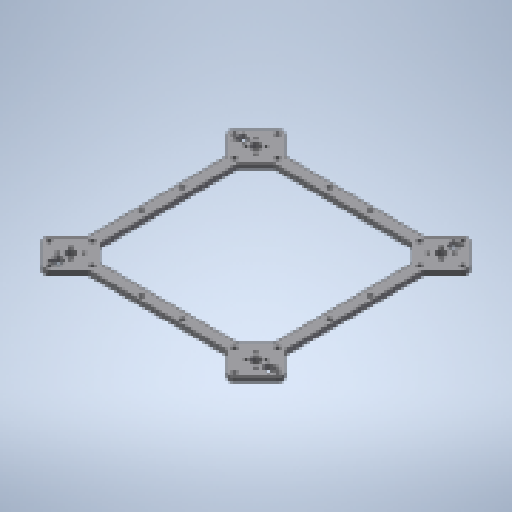
# Autodesk Inventor part: 终版
Saved by Autodesk Inventor 2025.2 (Build 292293000, 293)
## iProperties
Created: 2025-10-21
Part Number: 终版
Material: 常规
Document SubType Name: Modeling
Designer: BO‘S_SLAVE
Density: 1 g/cm^3
Appearance: 默认
Author: BO‘S_SLAVE
Autodesk Inventor part; units mm, degrees
ref_plane "YZ Plane" through (0, 0, 0) normal (1, 0, 0) x (0, 1, 0)
ref_plane "XZ Plane" through (0, 0, 0) normal (0, 1, 0) x (-1, 0, 0)
ref_plane "XY Plane" through (0, 0, 0) normal (0, 0, 1) x (1, 0, 0)
sketch "草图1" plane through (0, 0, 0) normal (0, 1, 0) x (-1, 0, 0)
  line L0 (0, 0) -> (-155.5635, 0)
  line L1 (-155.5635, 0) -> (-155.5635, -155.5635)
  line L2 (-155.5635, -155.5635) -> (0, -155.5635)
  line L3 (0, -155.5635) -> (0, 0)
  line L4 (0, 0) -> (-155.5635, -155.5635)
  line L5 (0, -155.5635) -> (-155.5635, 0)
  line L6 (5, 5) -> (-160.5635, 5)
  line L7 (-160.5635, 5) -> (-160.5635, -160.5635)
  line L8 (-160.5635, -160.5635) -> (5, -160.5635)
  line L9 (5, -160.5635) -> (5, 5)
  line L10 (-5, -5) -> (-150.5635, -5)
  line L11 (-150.5635, -5) -> (-150.5635, -150.5635)
  line L12 (-150.5635, -150.5635) -> (-5, -150.5635)
  line L13 (-5, -150.5635) -> (-5, -5)
  line L14 (0, 24.7487) -> (-24.7487, 0)
  line L15 (24.7487, 0) -> (0, 24.7487)
  line L16 (0, -24.7487) -> (24.7487, 0)
  line L17 (0, -24.7487) -> (-24.7487, 0)
  circle A0 centre (-94.7817, 1.109) radius 1.65
  circle A1 centre (-60.7817, 1.109) radius 1.65
  line L18 (0, -24.7487) -> (0, 24.7487)
  line L19 (-77.7817, -5) -> (-77.7817, 5)
  circle A2 centre (0, 0) radius 3.5
  circle A3 centre (-5.6569, -5.6569) radius 1.15
  circle A4 centre (5.6569, 5.6569) radius 1.15
  circle A5 centre (-4.2426, 4.2426) radius 1.15
  circle A6 centre (4.2426, -4.2426) radius 1.15
  line L20 (5.6569, 5.6569) -> (0, 0)
  line L21 (4.2426, -4.2426) -> (-4.2426, 4.2426)
  circle A7 centre (18, 0) radius 1.65
  line L22 (24.7487, 0) -> (0, 0)
  circle A8 centre (0, 18) radius 1.65
  circle A9 centre (-18, 0) radius 1.65
  circle A10 centre (0, -18) radius 1.65
  line L23 (-155.5635, 24.7487) -> (-180.3122, 0)
  line L24 (-130.8148, 0) -> (-155.5635, 24.7487)
  line L25 (-130.8148, 0) -> (-155.5635, -24.7487)
  line L26 (-180.3122, 0) -> (-155.5635, -24.7487)
  circle A11 centre (-173.5635, 0) radius 1.65
  circle A12 centre (-155.5635, 18) radius 1.65
  circle A13 centre (-137.5635, 0) radius 1.65
  circle A14 centre (-155.5635, -18) radius 1.65
  circle A15 centre (-159.8061, -4.2426) radius 1.15
  circle A16 centre (-151.3209, 4.2426) radius 1.15
  circle A17 centre (-161.2203, 5.6569) radius 1.15
  circle A18 centre (-155.5635, 0) radius 3.5
  circle A19 centre (-149.9066, -5.6569) radius 1.15
  line L27 (-180.3122, -155.5635) -> (-155.5635, -180.3122)
  line L28 (-155.5635, -130.8148) -> (-180.3122, -155.5635)
  line L29 (-155.5635, -130.8148) -> (-130.8148, -155.5635)
  line L30 (-155.5635, -180.3122) -> (-130.8148, -155.5635)
  circle A20 centre (-155.5635, -173.5635) radius 1.65
  circle A21 centre (-173.5635, -155.5635) radius 1.65
  circle A22 centre (-155.5635, -137.5635) radius 1.65
  circle A23 centre (-137.5635, -155.5635) radius 1.65
  circle A24 centre (-151.3209, -159.8061) radius 1.15
  circle A25 centre (-159.8061, -151.3209) radius 1.15
  circle A26 centre (-161.2203, -161.2203) radius 1.15
  circle A27 centre (-155.5635, -155.5635) radius 3.5
  circle A28 centre (-149.9066, -149.9066) radius 1.15
  line L31 (0, -180.3122) -> (24.7487, -155.5635)
  line L32 (-24.7487, -155.5635) -> (0, -180.3122)
  line L33 (-24.7487, -155.5635) -> (0, -130.8148)
  line L34 (24.7487, -155.5635) -> (0, -130.8148)
  circle A29 centre (18, -155.5635) radius 1.65
  circle A30 centre (0, -173.5635) radius 1.65
  circle A31 centre (-18, -155.5635) radius 1.65
  circle A32 centre (0, -137.5635) radius 1.65
  circle A33 centre (4.2426, -151.3209) radius 1.15
  circle A34 centre (-4.2426, -159.8061) radius 1.15
  circle A35 centre (5.6569, -161.2203) radius 1.15
  circle A36 centre (0, -155.5635) radius 3.5
  circle A37 centre (-5.6569, -149.9066) radius 1.15
  circle A38 centre (-156.6725, -94.7817) radius 1.65
  circle A39 centre (-156.6725, -60.7817) radius 1.65
  circle A40 centre (-60.7817, -156.6725) radius 1.65
  circle A41 centre (-94.7817, -156.6725) radius 1.65
  circle A42 centre (1.109, -60.7817) radius 1.65
  circle A43 centre (1.109, -94.7817) radius 1.65
  circle A44 centre (-60.7817, 1.1093) radius 1.65 projected
  circle A45 centre (-41.7817, -60.7817) radius 1.65 construction
  line L35 (-66.2817, -48.8909) -> (-66.2817, -106.6726) construction
  line L36 (-65.8148, -48.8909) -> (-66.2817, -48.8909) construction
  line L37 (-48.8909, -65.8148) -> (-65.8148, -48.8909) construction
  line L38 (-48.8909, -89.7487) -> (-48.8909, -65.8148) construction
  line L39 (-65.8148, -106.6726) -> (-48.8909, -89.7487) construction
  line L40 (-66.2817, -106.6726) -> (-65.8148, -106.6726) construction
  arc A46 (-61.6726, -28.8363) -> (-64.6726, -25.8363) centre (-64.6726, -28.8363) ccw construction
  line L41 (-61.6726, -35.8909) -> (-61.6726, -28.8363) construction
  arc A47 (-64.6726, -38.8909) -> (-61.6726, -35.8909) centre (-64.6726, -35.8909) ccw construction
  line L42 (-90.8909, -38.8909) -> (-64.6726, -38.8909) construction
  arc A48 (-93.8909, -35.8909) -> (-90.8909, -38.8909) centre (-90.8909, -35.8909) ccw construction
  line L43 (-93.8909, -28.8363) -> (-93.8909, -35.8909) construction
  arc A49 (-90.8909, -25.8363) -> (-93.8909, -28.8363) centre (-90.8909, -28.8363) ccw construction
  line L44 (-64.6726, -25.8363) -> (-90.8909, -25.8363) construction
  arc A50 (-115.3828, -60.3828) -> (-114.1807, -59.1807) centre (-113.7817, -60.7817) ccw construction
  line L45 (-114.1807, -59.1807) -> (-115.3828, -60.3828) construction
  circle A51 centre (-94.7817, -113.7817) radius 1.65 construction
  circle A52 centre (-155.5635, -137.5635) radius 1.65 construction
  line L46 (-157.9654, -162.7302) -> (-160.0223, -170.4065) construction
  line L47 (-153.1616, -162.7302) -> (-157.9654, -162.7302) construction
  line L48 (-151.1047, -170.4065) -> (-153.1616, -162.7302) construction
  line L49 (-160.0223, -170.4065) -> (-151.1047, -170.4065) construction
  circle A53 centre (-155.5635, -173.5635) radius 1.65 construction
  circle A54 centre (-137.5635, -155.5635) radius 1.65 construction
  circle A55 centre (-173.5635, -155.5635) radius 1.65 construction
  circle A56 centre (-151.3209, -159.8061) radius 1.15 construction
  circle A57 centre (-159.8061, -151.3209) radius 1.15 construction
  circle A58 centre (-161.2203, -161.2203) radius 1.15 construction
  arc A59 (-108.4906, -39.5876) -> (-107.7835, -37.8805) centre (-108.4906, -38.5876) ccw construction
  line L50 (-112.7333, -39.5876) -> (-108.4906, -39.5876) construction
  arc A60 (-113.4404, -39.2947) -> (-112.7333, -39.5876) centre (-112.7333, -38.5876) ccw construction
  line L51 (-115.683, -37.052) -> (-113.4404, -39.2947) construction
  arc A61 (-115.9759, -36.3449) -> (-115.683, -37.052) centre (-114.9759, -36.3449) ccw construction
  line L52 (-115.9759, -32.1023) -> (-115.9759, -36.3449) construction
  arc A62 (-114.2688, -31.3952) -> (-115.9759, -32.1023) centre (-114.9759, -32.1023) ccw construction
  line L53 (-107.7835, -37.8805) -> (-114.2688, -31.3952) construction
  arc A63 (-126.6328, -21.4454) -> (-125.9257, -19.7383) centre (-126.6328, -20.4454) ccw construction
  line L54 (-130.8754, -21.4454) -> (-126.6328, -21.4454) construction
  arc A64 (-131.5825, -21.1525) -> (-130.8754, -21.4454) centre (-130.8754, -20.4454) ccw construction
  line L55 (-133.8252, -18.9099) -> (-131.5825, -21.1525) construction
  arc A65 (-134.1181, -18.2028) -> (-133.8252, -18.9099) centre (-133.1181, -18.2028) ccw construction
  line L56 (-134.1181, -13.9602) -> (-134.1181, -18.2028) construction
  arc A66 (-132.4109, -13.253) -> (-134.1181, -13.9602) centre (-133.1181, -13.9602) ccw construction
  line L57 (-125.9257, -19.7383) -> (-132.4109, -13.253) construction
  arc A67 (-136.1181, -9.9602) -> (-136.4109, -9.253) centre (-137.1181, -9.9602) ccw construction
  line L58 (-136.1181, -14.2028) -> (-136.1181, -9.9602) construction
  arc A68 (-137.8252, -14.9099) -> (-136.1181, -14.2028) centre (-137.1181, -14.2028) ccw construction
  line L59 (-141.7749, -10.9602) -> (-137.8252, -14.9099) construction
  line L60 (-138.2394, -7.4246) -> (-141.7749, -10.9602) construction
  line L61 (-136.4109, -9.253) -> (-138.2394, -7.4246) construction
  arc A69 (-21.7383, -18.9099) -> (-21.4454, -18.2028) centre (-22.4454, -18.2028) ccw construction
  line L62 (-23.981, -21.1525) -> (-21.7383, -18.9099) construction
  arc A70 (-24.6881, -21.4454) -> (-23.981, -21.1525) centre (-24.6881, -20.4454) ccw construction
  line L63 (-28.9307, -21.4454) -> (-24.6881, -21.4454) construction
  arc A71 (-29.6378, -19.7383) -> (-28.9307, -21.4454) centre (-28.9307, -20.4454) ccw construction
  line L64 (-23.1525, -13.253) -> (-29.6378, -19.7383) construction
  arc A72 (-21.4454, -13.9602) -> (-23.1525, -13.253) centre (-22.4454, -13.9602) ccw construction
  line L65 (-21.4454, -18.2028) -> (-21.4454, -13.9602) construction
  arc A73 (-37.5876, -127.4612) -> (-37.2947, -128.1683) centre (-36.5876, -127.4612) ccw construction
  line L66 (-37.5876, -123.2186) -> (-37.5876, -127.4612) construction
  arc A74 (-35.8805, -122.5115) -> (-37.5876, -123.2186) centre (-36.5876, -123.2186) ccw construction
  line L67 (-27.981, -130.4109) -> (-35.8805, -122.5115) construction
  arc A75 (-28.6881, -132.1181) -> (-27.981, -130.4109) centre (-28.6881, -131.1181) ccw construction
  line L68 (-32.9307, -132.1181) -> (-28.6881, -132.1181) construction
  arc A76 (-33.6378, -131.8252) -> (-32.9307, -132.1181) centre (-32.9307, -131.1181) ccw construction
  line L69 (-37.2947, -128.1683) -> (-33.6378, -131.8252) construction
  arc A77 (-37.8805, -107.7835) -> (-39.5876, -108.4906) centre (-38.5876, -108.4906) ccw construction
  line L70 (-31.3952, -114.2688) -> (-37.8805, -107.7835) construction
  arc A78 (-32.1023, -115.9759) -> (-31.3952, -114.2688) centre (-32.1023, -114.9759) ccw construction
  line L71 (-36.3449, -115.9759) -> (-32.1023, -115.9759) construction
  arc A79 (-37.052, -115.683) -> (-36.3449, -115.9759) centre (-36.3449, -114.9759) ccw construction
  line L72 (-39.2947, -113.4404) -> (-37.052, -115.683) construction
  arc A80 (-39.5876, -112.7333) -> (-39.2947, -113.4404) centre (-38.5876, -112.7333) ccw construction
  line L73 (-39.5876, -108.4906) -> (-39.5876, -112.7333) construction
  arc A81 (-14.2028, -136.1181) -> (-14.9099, -137.8252) centre (-14.2028, -137.1181) ccw construction
  line L74 (-9.9602, -136.1181) -> (-14.2028, -136.1181) construction
  arc A82 (-9.253, -136.4109) -> (-9.9602, -136.1181) centre (-9.9602, -137.1181) ccw construction
  line L75 (-7.4246, -138.2394) -> (-9.253, -136.4109) construction
  line L76 (-10.9602, -141.7749) -> (-7.4246, -138.2394) construction
  line L77 (-14.9099, -137.8252) -> (-10.9602, -141.7749) construction
  arc A83 (-32.3449, -117.9759) -> (-33.052, -119.683) centre (-32.3449, -118.9759) ccw construction
  line L78 (-28.1023, -117.9759) -> (-32.3449, -117.9759) construction
  arc A84 (-27.3952, -118.2688) -> (-28.1023, -117.9759) centre (-28.1023, -118.9759) ccw construction
  line L79 (-23.7383, -121.9257) -> (-27.3952, -118.2688) construction
  arc A85 (-23.4454, -122.6328) -> (-23.7383, -121.9257) centre (-24.4454, -122.6328) ccw construction
  line L80 (-23.4454, -126.8754) -> (-23.4454, -122.6328) construction
  arc A86 (-25.1525, -127.5825) -> (-23.4454, -126.8754) centre (-24.4454, -126.8754) ccw construction
  line L81 (-33.052, -119.683) -> (-25.1525, -127.5825) construction
  line L82 (-18.617, -134.1181) -> (-13.9602, -134.1181) construction
  line L83 (-21.1525, -131.5825) -> (-18.617, -134.1181) construction
  arc A87 (-21.4454, -130.8754) -> (-21.1525, -131.5825) centre (-20.4454, -130.8754) ccw construction
  line L84 (-21.4454, -126.6328) -> (-21.4454, -130.8754) construction
  arc A88 (-19.7383, -125.9257) -> (-21.4454, -126.6328) centre (-20.4454, -126.6328) ccw construction
  line L85 (-13.253, -132.4109) -> (-19.7383, -125.9257) construction
  arc A89 (-13.9602, -134.1181) -> (-13.253, -132.4109) centre (-13.9602, -133.1181) ccw construction
  circle A90 centre (-4.2426, 4.2426) radius 1.15 construction
  circle A91 centre (4.2426, -4.2426) radius 1.15 construction
  circle A92 centre (0, 0) radius 3.5 construction
  circle A93 centre (-5.6569, -5.6569) radius 1.15 construction
  line L86 (4.4588, 14.843) -> (-4.4588, 14.843) construction
  line L87 (2.4019, 7.1667) -> (4.4588, 14.843) construction
  line L88 (-2.4019, 7.1667) -> (2.4019, 7.1667) construction
  line L89 (-4.4588, 14.843) -> (-2.4019, 7.1667) construction
  circle A94 centre (5.6569, 5.6569) radius 1.15 construction
  circle A95 centre (-18, 0) radius 1.65 construction
  circle A96 centre (0, -18) radius 1.65 construction
  circle A97 centre (0, 18) radius 1.65 construction
  circle A98 centre (18, 0) radius 1.65 construction
  circle A99 centre (-4.2426, -159.8061) radius 1.15 construction
  circle A100 centre (-5.6569, -149.9066) radius 1.15 construction
  circle A101 centre (4.2426, -151.3209) radius 1.15 construction
  line L90 (7.1667, -153.1616) -> (7.1667, -157.9654) construction
  line L91 (14.843, -151.1047) -> (7.1667, -153.1616) construction
  line L92 (14.843, -160.0223) -> (14.843, -151.1047) construction
  line L93 (7.1667, -157.9654) -> (14.843, -160.0223) construction
  circle A102 centre (0, -155.5635) radius 3.5 construction
  circle A103 centre (-18, -155.5635) radius 1.65 construction
  circle A104 centre (0, -173.5635) radius 1.65 construction
  circle A105 centre (18, -155.5635) radius 1.65 construction
  circle A106 centre (0, -137.5635) radius 1.65 construction
  circle A107 centre (5.6569, -161.2203) radius 1.15 construction
  arc A108 (-19.4454, -145.6033) -> (-19.1525, -146.3104) centre (-18.4454, -145.6033) ccw construction
  line L94 (-19.4454, -141.3607) -> (-19.4454, -145.6033) construction
  arc A109 (-17.7383, -140.6536) -> (-19.4454, -141.3607) centre (-18.4454, -141.3607) ccw construction
  line L95 (-13.7886, -144.6033) -> (-17.7383, -140.6536) construction
  line L96 (-17.3241, -148.1389) -> (-13.7886, -144.6033) construction
  line L97 (-19.1525, -146.3104) -> (-17.3241, -148.1389) construction
  arc A110 (-28.9307, -134.1181) -> (-29.6378, -135.8252) centre (-28.9307, -135.1181) ccw construction
  line L98 (-24.6881, -134.1181) -> (-28.9307, -134.1181) construction
  arc A111 (-23.981, -134.4109) -> (-24.6881, -134.1181) centre (-24.6881, -135.1181) ccw construction
  line L99 (-21.7383, -136.6536) -> (-23.981, -134.4109) construction
  arc A112 (-21.4454, -137.3607) -> (-21.7383, -136.6536) centre (-22.4454, -137.3607) ccw construction
  line L100 (-21.4454, -141.6033) -> (-21.4454, -137.3607) construction
  arc A113 (-23.1525, -142.3104) -> (-21.4454, -141.6033) centre (-22.4454, -141.6033) ccw construction
  line L101 (-29.6378, -135.8252) -> (-23.1525, -142.3104) construction
  arc A114 (-47.0729, -115.9759) -> (-47.78, -117.683) centre (-47.0729, -116.9759) ccw construction
  line L102 (-42.8302, -115.9759) -> (-47.0729, -115.9759) construction
  arc A115 (-42.1231, -116.2688) -> (-42.8302, -115.9759) centre (-42.8302, -116.9759) ccw construction
  line L103 (-39.8805, -118.5115) -> (-42.1231, -116.2688) construction
  arc A116 (-39.5876, -119.2186) -> (-39.8805, -118.5115) centre (-40.5876, -119.2186) ccw construction
  line L104 (-39.5876, -123.4612) -> (-39.5876, -119.2186) construction
  arc A117 (-41.2947, -124.1683) -> (-39.5876, -123.4612) centre (-40.5876, -123.4612) ccw construction
  line L105 (-47.78, -117.683) -> (-41.2947, -124.1683) construction
  circle A118 centre (-60.7817, -41.7817) radius 1.65 construction
  circle A119 centre (-94.7817, -41.7817) radius 1.65 construction
  arc A120 (-28.1023, -37.5876) -> (-27.3952, -37.2947) centre (-28.1023, -36.5876) ccw construction
  line L106 (-32.3449, -37.5876) -> (-28.1023, -37.5876) construction
  arc A121 (-33.052, -35.8805) -> (-32.3449, -37.5876) centre (-32.3449, -36.5876) ccw construction
  line L107 (-25.1525, -27.981) -> (-33.052, -35.8805) construction
  arc A122 (-23.4454, -28.6881) -> (-25.1525, -27.981) centre (-24.4454, -28.6881) ccw construction
  line L108 (-23.4454, -32.9307) -> (-23.4454, -28.6881) construction
  arc A123 (-23.7383, -33.6378) -> (-23.4454, -32.9307) centre (-24.4454, -32.9307) ccw construction
  line L109 (-27.3952, -37.2947) -> (-23.7383, -33.6378) construction
  arc A124 (-19.1525, -9.253) -> (-19.4454, -9.9602) centre (-18.4454, -9.9602) ccw construction
  line L110 (-17.3241, -7.4246) -> (-19.1525, -9.253) construction
  line L111 (-13.7886, -10.9602) -> (-17.3241, -7.4246) construction
  line L112 (-17.7383, -14.9099) -> (-13.7886, -10.9602) construction
  arc A125 (-19.4454, -14.2028) -> (-17.7383, -14.9099) centre (-18.4454, -14.2028) ccw construction
  line L113 (-19.4454, -9.9602) -> (-19.4454, -14.2028) construction
  arc A126 (-37.2947, -27.3952) -> (-37.5876, -28.1023) centre (-36.5876, -28.1023) ccw construction
  line L114 (-33.6378, -23.7383) -> (-37.2947, -27.3952) construction
  arc A127 (-32.9307, -23.4454) -> (-33.6378, -23.7383) centre (-32.9307, -24.4454) ccw construction
  line L115 (-28.6881, -23.4454) -> (-32.9307, -23.4454) construction
  arc A128 (-27.981, -25.1525) -> (-28.6881, -23.4454) centre (-28.6881, -24.4454) ccw construction
  line L116 (-35.8805, -33.052) -> (-27.981, -25.1525) construction
  arc A129 (-37.5876, -32.3449) -> (-35.8805, -33.052) centre (-36.5876, -32.3449) ccw construction
  line L117 (-37.5876, -28.1023) -> (-37.5876, -32.3449) construction
  arc A130 (-47.78, -37.8805) -> (-47.0729, -39.5876) centre (-47.0729, -38.5876) ccw construction
  line L118 (-41.2947, -31.3952) -> (-47.78, -37.8805) construction
  arc A131 (-39.5876, -32.1023) -> (-41.2947, -31.3952) centre (-40.5876, -32.1023) ccw construction
  line L119 (-39.5876, -36.3449) -> (-39.5876, -32.1023) construction
  arc A132 (-39.8805, -37.052) -> (-39.5876, -36.3449) centre (-40.5876, -36.3449) ccw construction
  line L120 (-42.1231, -39.2947) -> (-39.8805, -37.052) construction
  arc A133 (-42.8302, -39.5876) -> (-42.1231, -39.2947) centre (-42.8302, -38.5876) ccw construction
  line L121 (-47.0729, -39.5876) -> (-42.8302, -39.5876) construction
  arc A134 (-9.9602, -19.4454) -> (-9.253, -19.1525) centre (-9.9602, -18.4454) ccw construction
  line L122 (-14.2028, -19.4454) -> (-9.9602, -19.4454) construction
  arc A135 (-14.9099, -17.7383) -> (-14.2028, -19.4454) centre (-14.2028, -18.4454) ccw construction
  line L123 (-10.9602, -13.7886) -> (-14.9099, -17.7383) construction
  line L124 (-7.4246, -17.3241) -> (-10.9602, -13.7886) construction
  line L125 (-9.253, -19.1525) -> (-7.4246, -17.3241) construction
  arc A136 (-21.4454, -28.9307) -> (-19.7383, -29.6378) centre (-20.4454, -28.9307) ccw construction
  line L126 (-21.4454, -24.6881) -> (-21.4454, -28.9307) construction
  arc A137 (-21.1525, -23.981) -> (-21.4454, -24.6881) centre (-20.4454, -24.6881) ccw construction
  line L127 (-18.9099, -21.7383) -> (-21.1525, -23.981) construction
  arc A138 (-18.2028, -21.4454) -> (-18.9099, -21.7383) centre (-18.2028, -22.4454) ccw construction
  line L128 (-13.9602, -21.4454) -> (-18.2028, -21.4454) construction
  arc A139 (-13.253, -23.1525) -> (-13.9602, -21.4454) centre (-13.9602, -22.4454) ccw construction
  line L129 (-19.7383, -29.6378) -> (-13.253, -23.1525) construction
  arc A140 (-39.5876, -47.0729) -> (-37.8805, -47.78) centre (-38.5876, -47.0729) ccw construction
  line L130 (-39.5876, -42.8302) -> (-39.5876, -47.0729) construction
  arc A141 (-39.2947, -42.1231) -> (-39.5876, -42.8302) centre (-38.5876, -42.8302) ccw construction
  line L131 (-37.052, -39.8805) -> (-39.2947, -42.1231) construction
  arc A142 (-36.3449, -39.5876) -> (-37.052, -39.8805) centre (-36.3449, -40.5876) ccw construction
  line L132 (-32.1023, -39.5876) -> (-36.3449, -39.5876) construction
  arc A143 (-31.3952, -41.2947) -> (-32.1023, -39.5876) centre (-32.1023, -40.5876) ccw construction
  line L133 (-37.8805, -47.78) -> (-31.3952, -41.2947) construction
  arc A144 (-136.6536, -21.7383) -> (-137.3607, -21.4454) centre (-137.3607, -22.4454) ccw construction
  line L134 (-134.4109, -23.981) -> (-136.6536, -21.7383) construction
  arc A145 (-134.1181, -24.6881) -> (-134.4109, -23.981) centre (-135.1181, -24.6881) ccw construction
  line L135 (-134.1181, -28.9307) -> (-134.1181, -24.6881) construction
  arc A146 (-135.8252, -29.6378) -> (-134.1181, -28.9307) centre (-135.1181, -28.9307) ccw construction
  line L136 (-142.3104, -23.1525) -> (-135.8252, -29.6378) construction
  arc A147 (-141.6033, -21.4454) -> (-142.3104, -23.1525) centre (-141.6033, -22.4454) ccw construction
  line L137 (-137.3607, -21.4454) -> (-141.6033, -21.4454) construction
  line L138 (-162.7302, -2.4019) -> (-162.7302, 2.4019) construction
  line L139 (-170.4065, -4.4588) -> (-162.7302, -2.4019) construction
  line L140 (-170.4065, 4.4588) -> (-170.4065, -4.4588) construction
  line L141 (-162.7302, 2.4019) -> (-170.4065, 4.4588) construction
  circle A148 centre (-155.5635, 18) radius 1.65 construction
  circle A149 centre (-173.5635, 0) radius 1.65 construction
  circle A150 centre (-137.5635, 0) radius 1.65 construction
  circle A151 centre (-155.5635, -18) radius 1.65 construction
  circle A152 centre (-161.2203, 5.6569) radius 1.15 construction
  circle A153 centre (-149.9066, -5.6569) radius 1.15 construction
  circle A154 centre (-155.5635, 0) radius 3.5 construction
  circle A155 centre (-151.3209, 4.2426) radius 1.15 construction
  circle A156 centre (-159.8061, -4.2426) radius 1.15 construction
  arc A157 (-146.3104, -19.1525) -> (-145.6033, -19.4454) centre (-145.6033, -18.4454) ccw construction
  line L142 (-148.1389, -17.3241) -> (-146.3104, -19.1525) construction
  line L143 (-144.6033, -13.7886) -> (-148.1389, -17.3241) construction
  line L144 (-140.6536, -17.7383) -> (-144.6033, -13.7886) construction
  arc A158 (-141.3607, -19.4454) -> (-140.6536, -17.7383) centre (-141.3607, -18.4454) ccw construction
  line L145 (-145.6033, -19.4454) -> (-141.3607, -19.4454) construction
  arc A159 (-128.1683, -37.2947) -> (-127.4612, -37.5876) centre (-127.4612, -36.5876) ccw construction
  line L146 (-131.8252, -33.6378) -> (-128.1683, -37.2947) construction
  arc A160 (-132.1181, -32.9307) -> (-131.8252, -33.6378) centre (-131.1181, -32.9307) ccw construction
  line L147 (-132.1181, -28.6881) -> (-132.1181, -32.9307) construction
  arc A161 (-130.4109, -27.981) -> (-132.1181, -28.6881) centre (-131.1181, -28.6881) ccw construction
  line L148 (-122.5115, -35.8805) -> (-130.4109, -27.981) construction
  arc A162 (-123.2186, -37.5876) -> (-122.5115, -35.8805) centre (-123.2186, -36.5876) ccw construction
  line L149 (-127.4612, -37.5876) -> (-123.2186, -37.5876) construction
  arc A163 (-117.683, -47.78) -> (-115.9759, -47.0729) centre (-116.9759, -47.0729) ccw construction
  line L150 (-124.1683, -41.2947) -> (-117.683, -47.78) construction
  arc A164 (-123.4612, -39.5876) -> (-124.1683, -41.2947) centre (-123.4612, -40.5876) ccw construction
  line L151 (-119.2186, -39.5876) -> (-123.4612, -39.5876) construction
  arc A165 (-118.5115, -39.8805) -> (-119.2186, -39.5876) centre (-119.2186, -40.5876) ccw construction
  line L152 (-116.2688, -42.1231) -> (-118.5115, -39.8805) construction
  arc A166 (-115.9759, -42.8302) -> (-116.2688, -42.1231) centre (-116.9759, -42.8302) ccw construction
  line L153 (-115.9759, -47.0729) -> (-115.9759, -42.8302) construction
  arc A167 (-117.9759, -28.1023) -> (-118.2688, -27.3952) centre (-118.9759, -28.1023) ccw construction
  line L154 (-117.9759, -32.3449) -> (-117.9759, -28.1023) construction
  arc A168 (-119.683, -33.052) -> (-117.9759, -32.3449) centre (-118.9759, -32.3449) ccw construction
  line L155 (-127.5825, -25.1525) -> (-119.683, -33.052) construction
  arc A169 (-126.8754, -23.4454) -> (-127.5825, -25.1525) centre (-126.8754, -24.4454) ccw construction
  line L156 (-122.6328, -23.4454) -> (-126.8754, -23.4454) construction
  arc A170 (-121.9257, -23.7383) -> (-122.6328, -23.4454) centre (-122.6328, -24.4454) ccw construction
  line L157 (-118.2688, -27.3952) -> (-121.9257, -23.7383) construction
  arc A171 (-119.2186, -115.9759) -> (-118.5115, -115.683) centre (-119.2186, -114.9759) ccw construction
  line L158 (-123.4612, -115.9759) -> (-119.2186, -115.9759) construction
  arc A172 (-124.1683, -114.2688) -> (-123.4612, -115.9759) centre (-123.4612, -114.9759) ccw construction
  line L159 (-117.683, -107.7835) -> (-124.1683, -114.2688) construction
  arc A173 (-115.9759, -108.4906) -> (-117.683, -107.7835) centre (-116.9759, -108.4906) ccw construction
  line L160 (-115.9759, -112.7333) -> (-115.9759, -108.4906) construction
  arc A174 (-116.2688, -113.4404) -> (-115.9759, -112.7333) centre (-116.9759, -112.7333) ccw construction
  line L161 (-118.5115, -115.683) -> (-116.2688, -113.4404) construction
  arc A175 (-132.1181, -126.8754) -> (-130.4109, -127.5825) centre (-131.1181, -126.8754) ccw construction
  line L162 (-132.1181, -122.6328) -> (-132.1181, -126.8754) construction
  arc A176 (-131.8252, -121.9257) -> (-132.1181, -122.6328) centre (-131.1181, -122.6328) ccw construction
  line L163 (-127.8754, -117.9759) -> (-131.8252, -121.9257) construction
  line L164 (-123.2186, -117.9759) -> (-127.8754, -117.9759) construction
  arc A177 (-122.5115, -119.683) -> (-123.2186, -117.9759) centre (-123.2186, -118.9759) ccw construction
  line L165 (-130.4109, -127.5825) -> (-122.5115, -119.683) construction
  arc A178 (-137.3607, -134.1181) -> (-136.6536, -133.8252) centre (-137.3607, -133.1181) ccw construction
  line L166 (-141.6033, -134.1181) -> (-137.3607, -134.1181) construction
  arc A179 (-142.3104, -132.4109) -> (-141.6033, -134.1181) centre (-141.6033, -133.1181) ccw construction
  line L167 (-135.8252, -125.9257) -> (-142.3104, -132.4109) construction
  arc A180 (-134.1181, -126.6328) -> (-135.8252, -125.9257) centre (-135.1181, -126.6328) ccw construction
  line L168 (-134.1181, -130.8754) -> (-134.1181, -126.6328) construction
  arc A181 (-134.4109, -131.5825) -> (-134.1181, -130.8754) centre (-135.1181, -130.8754) ccw construction
  line L169 (-136.6536, -133.8252) -> (-134.4109, -131.5825) construction
  arc A182 (-134.1181, -141.6033) -> (-132.4109, -142.3104) centre (-133.1181, -141.6033) ccw construction
  line L170 (-134.1181, -137.3607) -> (-134.1181, -141.6033) construction
  arc A183 (-133.8252, -136.6536) -> (-134.1181, -137.3607) centre (-133.1181, -137.3607) ccw construction
  line L171 (-131.5825, -134.4109) -> (-133.8252, -136.6536) construction
  arc A184 (-130.8754, -134.1181) -> (-131.5825, -134.4109) centre (-130.8754, -135.1181) ccw construction
  line L172 (-126.6328, -134.1181) -> (-130.8754, -134.1181) construction
  arc A185 (-125.9257, -135.8252) -> (-126.6328, -134.1181) centre (-126.6328, -135.1181) ccw construction
  line L173 (-132.4109, -142.3104) -> (-125.9257, -135.8252) construction
  arc A186 (-107.7835, -117.683) -> (-108.4906, -115.9759) centre (-108.4906, -116.9759) ccw construction
  line L174 (-114.2688, -124.1683) -> (-107.7835, -117.683) construction
  arc A187 (-115.9759, -123.4612) -> (-114.2688, -124.1683) centre (-114.9759, -123.4612) ccw construction
  line L175 (-115.9759, -119.2186) -> (-115.9759, -123.4612) construction
  arc A188 (-115.683, -118.5115) -> (-115.9759, -119.2186) centre (-114.9759, -119.2186) ccw construction
  line L176 (-113.4404, -116.2688) -> (-115.683, -118.5115) construction
  arc A189 (-112.7333, -115.9759) -> (-113.4404, -116.2688) centre (-112.7333, -116.9759) ccw construction
  line L177 (-108.4906, -115.9759) -> (-112.7333, -115.9759) construction
  arc A190 (-122.6328, -132.1181) -> (-121.9257, -131.8252) centre (-122.6328, -131.1181) ccw construction
  line L178 (-126.8754, -132.1181) -> (-122.6328, -132.1181) construction
  arc A191 (-127.5825, -130.4109) -> (-126.8754, -132.1181) centre (-126.8754, -131.1181) ccw construction
  line L179 (-119.683, -122.5115) -> (-127.5825, -130.4109) construction
  arc A192 (-117.9759, -123.2186) -> (-119.683, -122.5115) centre (-118.9759, -123.2186) ccw construction
  line L180 (-117.9759, -127.4612) -> (-117.9759, -123.2186) construction
  arc A193 (-118.2688, -128.1683) -> (-117.9759, -127.4612) centre (-118.9759, -127.4612) ccw construction
  line L181 (-121.9257, -131.8252) -> (-118.2688, -128.1683) construction
  line L182 (-141.7749, -144.6033) -> (-138.2394, -148.1389) construction
  line L183 (-137.8252, -140.6536) -> (-141.7749, -144.6033) construction
  arc A194 (-136.1181, -141.3607) -> (-137.8252, -140.6536) centre (-137.1181, -141.3607) ccw construction
  line L184 (-136.1181, -145.6033) -> (-136.1181, -141.3607) construction
  arc A195 (-136.4109, -146.3104) -> (-136.1181, -145.6033) centre (-137.1181, -145.6033) ccw construction
  line L185 (-138.2394, -148.1389) -> (-136.4109, -146.3104) construction
  line L186 (-144.6033, -141.7749) -> (-140.6536, -137.8252) construction
  line L187 (-148.1389, -138.2394) -> (-144.6033, -141.7749) construction
  line L188 (-146.3104, -136.4109) -> (-148.1389, -138.2394) construction
  arc A196 (-145.6033, -136.1181) -> (-146.3104, -136.4109) centre (-145.6033, -137.1181) ccw construction
  line L189 (-141.3607, -136.1181) -> (-145.6033, -136.1181) construction
  arc A197 (-140.6536, -137.8252) -> (-141.3607, -136.1181) centre (-141.3607, -137.1181) ccw construction
  circle A198 centre (-149.9066, -149.9066) radius 1.15 construction
  circle A199 centre (-155.5635, -155.5635) radius 3.5 construction
  line L190 (-84.2817, -106.6726) -> (-71.2817, -106.6726) construction
  line L191 (-84.2817, -48.8909) -> (-84.2817, -106.6726) construction
  line L192 (-71.2817, -48.8909) -> (-84.2817, -48.8909) construction
  line L193 (-71.2817, -106.6726) -> (-71.2817, -48.8909) construction
  line L194 (-61.6726, -116.6726) -> (-90.8909, -116.6726) construction
  line L195 (-61.6726, -129.7817) -> (-61.6726, -116.6726) construction
  arc A200 (-64.6726, -132.7817) -> (-61.6726, -129.7817) centre (-64.6726, -129.7817) ccw construction
  line L196 (-90.8909, -132.7817) -> (-64.6726, -132.7817) construction
  arc A201 (-93.8909, -129.7817) -> (-90.8909, -132.7817) centre (-90.8909, -129.7817) ccw construction
  line L197 (-93.8909, -119.6726) -> (-93.8909, -129.7817) construction
  arc A202 (-90.8909, -116.6726) -> (-93.8909, -119.6726) centre (-90.8909, -119.6726) ccw construction
  circle A203 centre (-60.7817, -113.7817) radius 1.65 construction
  circle A204 centre (-41.7817, -94.7817) radius 1.65 construction
  arc A205 (-64.6726, -20.8363) -> (-61.6726, -17.8363) centre (-64.6726, -17.8363) ccw construction
  line L198 (-90.8909, -20.8363) -> (-64.6726, -20.8363) construction
  arc A206 (-93.8909, -17.8363) -> (-90.8909, -20.8363) centre (-90.8909, -17.8363) ccw construction
  line L199 (-93.8909, -15.7817) -> (-93.8909, -17.8363) construction
  arc A207 (-90.8909, -12.7817) -> (-93.8909, -15.7817) centre (-90.8909, -15.7817) ccw construction
  line L200 (-64.6726, -12.7817) -> (-90.8909, -12.7817) construction
  arc A208 (-61.6726, -15.7817) -> (-64.6726, -12.7817) centre (-64.6726, -15.7817) ccw construction
  line L201 (-61.6726, -17.8363) -> (-61.6726, -15.7817) construction
  line L202 (-89.2817, -106.6726) -> (-89.2817, -48.8909) construction
  line L203 (-89.7487, -106.6726) -> (-89.2817, -106.6726) construction
  line L204 (-106.6726, -89.7487) -> (-89.7487, -106.6726) construction
  line L205 (-106.6726, -65.8148) -> (-106.6726, -89.7487) construction
  line L206 (-89.7487, -48.8909) -> (-106.6726, -65.8148) construction
  line L207 (-89.2817, -48.8909) -> (-89.7487, -48.8909) construction
  circle A209 centre (-113.7817, -94.7817) radius 1.65 construction
  arc A210 (-56.6726, -9.7817) -> (-58.6726, -7.7817) centre (-58.6726, -9.7817) ccw construction
  line L208 (-96.8909, -7.7817) -> (-58.6726, -7.7817) construction
  arc A211 (-96.8909, -7.7817) -> (-98.8909, -9.7817) centre (-96.8909, -9.7817) ccw construction
  line L209 (-98.8909, -35.2878) -> (-98.8909, -9.7817) construction
  arc A212 (-104.0122, -37.4092) -> (-98.8909, -35.2878) centre (-101.8909, -35.2878) ccw construction
  line L210 (-136.1181, -5.3033) -> (-104.0122, -37.4092) construction
  line L211 (-134.3503, -3.5355) -> (-136.1181, -5.3033) construction
  arc A213 (-134.3503, -3.5355) -> (-134.3503, 3.5355) centre (-137.8858, 0) ccw construction
  line L212 (-152.028, 21.2132) -> (-134.3503, 3.5355) construction
  arc A214 (-152.028, 21.2132) -> (-159.099, 21.2132) centre (-155.5635, 17.6777) ccw construction
  line L213 (-176.7767, 3.5355) -> (-159.099, 21.2132) construction
  arc A215 (-176.7767, 3.5355) -> (-176.7767, -3.5355) centre (-173.2412, 0) ccw construction
  line L214 (-159.099, -21.2132) -> (-176.7767, -3.5355) construction
  arc A216 (-159.099, -21.2132) -> (-152.028, -21.2132) centre (-155.5635, -17.6777) ccw construction
  line L215 (-150.2602, -19.4454) -> (-152.028, -21.2132) construction
  line L216 (-116.6726, -53.033) -> (-150.2602, -19.4454) construction
  line L217 (-116.6726, -102.5305) -> (-116.6726, -53.033) construction
  line L218 (-150.2602, -136.1181) -> (-116.6726, -102.5305) construction
  line L219 (-152.028, -134.3503) -> (-150.2602, -136.1181) construction
  arc A217 (-152.028, -134.3503) -> (-159.099, -134.3503) centre (-155.5635, -137.8858) ccw construction
  line L220 (-176.7767, -152.028) -> (-159.099, -134.3503) construction
  arc A218 (-176.7767, -152.028) -> (-176.7767, -159.099) centre (-173.2412, -155.5635) ccw construction
  line L221 (-159.099, -176.7767) -> (-176.7767, -159.099) construction
  arc A219 (-159.099, -176.7767) -> (-152.028, -176.7767) centre (-155.5635, -173.2412) ccw construction
  line L222 (-134.3503, -159.099) -> (-152.028, -176.7767) construction
  arc A220 (-134.3503, -159.099) -> (-134.3503, -152.028) centre (-137.8858, -155.5635) ccw construction
  line L223 (-136.1181, -150.2602) -> (-134.3503, -152.028) construction
  line L224 (-104.0122, -118.1543) -> (-136.1181, -150.2602) construction
  arc A221 (-98.8909, -120.2756) -> (-104.0122, -118.1543) centre (-101.8909, -120.2756) ccw construction
  line L225 (-98.8909, -137.7817) -> (-98.8909, -120.2756) construction
  line L226 (-56.6726, -137.7817) -> (-98.8909, -137.7817) construction
  line L227 (-56.6726, -120.2756) -> (-56.6726, -137.7817) construction
  arc A222 (-51.5513, -118.1543) -> (-56.6726, -120.2756) centre (-53.6726, -120.2756) ccw construction
  line L228 (-19.4454, -150.2602) -> (-51.5513, -118.1543) construction
  line L229 (-21.2132, -152.028) -> (-19.4454, -150.2602) construction
  arc A223 (-21.2132, -152.028) -> (-21.2132, -159.099) centre (-17.6777, -155.5635) ccw construction
  line L230 (-3.5355, -176.7767) -> (-21.2132, -159.099) construction
  arc A224 (-3.5355, -176.7767) -> (3.5355, -176.7767) centre (0, -173.2412) ccw construction
  line L231 (21.2132, -159.099) -> (3.5355, -176.7767) construction
  arc A225 (21.2132, -159.099) -> (21.2132, -152.028) centre (17.6777, -155.5635) ccw construction
  line L232 (3.5355, -134.3503) -> (21.2132, -152.028) construction
  arc A226 (3.5355, -134.3503) -> (-3.5355, -134.3503) centre (0, -137.8858) ccw construction
  line L233 (-5.3033, -136.1181) -> (-3.5355, -134.3503) construction
  line L234 (-38.8909, -102.5305) -> (-5.3033, -136.1181) construction
  line L235 (-38.8909, -53.033) -> (-38.8909, -102.5305) construction
  line L236 (-5.3033, -19.4454) -> (-38.8909, -53.033) construction
  line L237 (-3.5355, -21.2132) -> (-5.3033, -19.4454) construction
  arc A227 (-3.5355, -21.2132) -> (3.5355, -21.2132) centre (0, -17.6777) ccw construction
  line L238 (21.2132, -3.5355) -> (3.5355, -21.2132) construction
  arc A228 (21.2132, -3.5355) -> (21.2132, 3.5355) centre (17.6777, 0) ccw construction
  line L239 (3.5355, 21.2132) -> (21.2132, 3.5355) construction
  arc A229 (3.5355, 21.2132) -> (-3.5355, 21.2132) centre (0, 17.6777) ccw construction
  line L240 (-21.2132, 3.5355) -> (-3.5355, 21.2132) construction
  arc A230 (-21.2132, 3.5355) -> (-21.2132, -3.5355) centre (-17.6777, 0) ccw construction
  line L241 (-19.4454, -5.3033) -> (-21.2132, -3.5355) construction
  line L242 (-51.5513, -37.4092) -> (-19.4454, -5.3033) construction
  arc A231 (-56.6726, -35.2878) -> (-51.5513, -37.4092) centre (-53.6726, -35.2878) ccw construction
  line L243 (-56.6726, -9.7817) -> (-56.6726, -35.2878) construction
  line L244 (-2.4019, 7.1667) -> (-4.4588, 14.843)
  line L245 (4.4588, 14.843) -> (-4.4588, 14.843)
  line L246 (2.4019, 7.1667) -> (4.4588, 14.843)
  line L247 (-2.4019, 7.1667) -> (2.4019, 7.1667)
  line L248 (-162.7302, -2.4019) -> (-170.4065, -4.4588)
  line L249 (-162.7302, -2.4019) -> (-162.7302, 2.4019)
  line L250 (-170.4065, 4.4588) -> (-170.4065, -4.4588)
  line L251 (-162.7302, 2.4019) -> (-170.4065, 4.4588)
  line L252 (-153.1616, -162.7302) -> (-151.1047, -170.4065)
  line L253 (-153.1616, -162.7302) -> (-157.9654, -162.7302)
  line L254 (-160.0223, -170.4065) -> (-151.1047, -170.4065)
  line L255 (-157.9654, -162.7302) -> (-160.0223, -170.4065)
  line L256 (7.1667, -153.1616) -> (14.843, -151.1047)
  line L257 (7.1667, -153.1616) -> (7.1667, -157.9654)
  line L258 (14.843, -160.0223) -> (14.843, -151.1047)
  line L259 (7.1667, -157.9654) -> (14.843, -160.0223)
  point P0 (-77.7817, -77.7817)
  point P1 (-19.7487, 5)
  point P2 (5, -19.7487)
  point P3 (-12.3744, -12.3744)
  point P4 (-77.7817, -77.7817)
  point P5 (-143.1891, -12.3744)
  point P6 (-135.8148, -5)
  point P7 (-19.7487, -5)
  point P8 (-19.7487, -150.5635)
  point P9 (-135.8148, -150.5635)
  point P10 (-150.5635, -135.8148)
  point P11 (-150.5635, -19.7487)
  point P12 (-5, -19.7487)
  point P13 (-5, -135.8148)
  point P14 (4.7129, 5)
  point P15 (5, 4.7129)
  point P16 (-135.8148, 5)
  point P17 (-160.5635, -19.7487)
  point P18 (-160.5635, -135.8148)
  point P19 (-135.8148, -160.5635)
  point P20 (-19.7487, -160.5635)
  point P21 (5, -135.8148)
  point P22 (5, -160.2764)
  point P23 (4.7129, -160.5635)
  point P24 (-160.2764, -160.5635)
  point P25 (-160.5635, -160.2764)
  point P26 (-160.5635, 4.7129)
  point P27 (-160.2764, 5)
  point P28 (-5.108, 5)
  point P29 (-3.3772, 5)
  dimension "d0" = 220
  dimension "d1" = 45
  dimension "d21" = 35
  dimension "d22" = 35
  dimension "d28" = 3.3
  dimension "d29" = 3.3
  dimension "d46" = 5
  dimension "d47" = 5
  dimension "d48" = 5
  dimension "d49" = 5
  dimension "d50" = 17
  dimension "d51" = 17
  dimension "d74" = 7
  dimension "d75" = 2.3
  dimension "d76" = 2.3
  dimension "d77" = 2.3
  dimension "d78" = 2.3
  dimension "d79" = 8
  dimension "d80" = 8
  dimension "d81" = 12
  dimension "d82" = 3.3
  dimension "d83" = 18
  dimension "d86" = 360
  dimension "d90" = 360
  dimension "d94" = 360
  dimension "d97" = 6.109
  dimension "d98" = 6.109
  dimension "d101" = 360
  constraints: 94 end point, 44 centre point, 7 point on line, 6 collinear, 6 parallel, 6 perpendicular, 5 midpoint, 3 horizontal, 2 coincident, 178 other
  measures "d0" distance of L2.end L0.end
  measures "d1" angle of L3 L5
  measures "d21" distance of L14.start L14.end
  measures "d22" distance of L15.start L14.start
  measures "d28" diameter of A0
  measures "d29" diameter of A1
  measures "d46" distance between parallel lines of L1 L11
  measures "d47" distance between parallel lines of L1 L7
  measures "d48" distance between parallel lines of L10 L0
  measures "d49" distance between parallel lines of L0 L6
  measures "d50" distance from line of L19 A0.centre
  measures "d51" distance from line of L19 A1.centre
  measures "d74" diameter of A2
  measures "d75" diameter of A3
  measures "d76" diameter of A4
  measures "d77" diameter of A5
  measures "d78" diameter of A6
  measures "d79" distance of A3.centre L20.end
  measures "d80" distance of A4.centre L0.start
  measures "d81" distance of L21.start L21.end
  measures "d82" diameter of A7
  measures "d83" distance of L0.start A7.centre
  measures "d97" distance from line of L10 A0.centre
  measures "d98" distance from line of L10 A1.centre
extrude "拉伸1" add sketch "草图1" along normal blind 4 contours L25 L10 A19 L5 A18 L0 A13 | L24 L6 L19 L0 A0 | L0 A13 A18 L1 A14 L26 L7 A15 A17 L6 A16 L24 | L0 A0 L19 L10 L25 | L6 A16 A17 L7 A15 L26 L23 L24 | L25 L5 A19 L10 | L6 L14 L0 A1 L19 | L19 L0 A1 L17 L10 | L25 L11 A19 L5 | L14 L18 A8 L245 L244 L247 L6 A5 | L6 A5 L21 A2 L0 A9 L14 | L17 L0 A9 A2 L4 A3 L10 | L10 A3 L4 L17 | A19 L11 L25 L1 A14 A18 L5 | L11 L29 L1 A38 A39 L25 | L15 L22 A7 L9 A4 L6 L18 L247 L246 L245 A8 | L26 L1 A39 A38 L28 L7 | L4 A3 L13 L17 | L29 L12 A28 L4 | L4 A28 L11 L29 | L33 L13 A37 L5 | L5 A37 L12 L33 | L11 A28 L4 A27 L1 A22 L29 | L6 L18 A2 L21 A5 | L16 L9 A6 L22 A7 | L28 L1 A22 A27 L2 A23 L30 L8 A24 A26 L7 A25 | L7 A25 A26 L8 A24 L30 L27 L28 | L4 A2 L3 A10 L17 L13 A3 | L17 L3 A42 A43 L33 L13 | L29 L2 A23 A27 L4 A28 L12 | L12 L33 L2 A40 A41 L29 | L12 A37 L5 A36 L2 A31 L33 | L33 L3 A32 A36 L5 A37 L13 | L6 A4 L20 A2 L18 | L16 L3 A10 A2 L21 A6 L9 | L9 L34 L3 A43 A42 L16 | L2 A41 A40 L32 L8 L30 | L2 A31 A36 L3 A32 L34 L9 A33 A35 L8 A34 L32 | L34 L31 L32 L8 A34 A35 L9 A33 | A4 L9 L22 A2 L20 | A2 L22 L9 A6 L21
fillet "圆角1" radius 5 8 edges at (180.3122, 2, 0) (155.5635, 2, 24.7487) (0, 2, 24.7487) (-24.7487, 2, 0) (-24.7487, 2, -155.5635) (0, 2, -180.3122) (155.5635, 2, -180.3122) (180.3122, 2, -155.5635)
